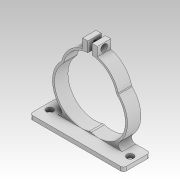
# Autodesk Inventor part: MotorTestBracket
Saved by Autodesk Inventor 2020 (Build 240168000, 168)
## iProperties
Created: 2022-01-15
Part Number: MotorTestBracket
Material: Generic
Document SubType Name: Modeling
Designer: DDeGo
Density: 1 g/cm^3
Appearance: Default
Author: DDeGo
Autodesk Inventor part; units mm, degrees
ref_plane "YZ Plane" through (0, 0, 0) normal (1, 0, 0) x (0, 1, 0)
ref_plane "XZ Plane" through (0, 0, 0) normal (0, 1, 0) x (-1, 0, 0)
ref_plane "XY Plane" through (0, 0, 0) normal (0, 0, 1) x (1, 0, 0)
sketch "Block1" plane through (0, 0, 0) normal (0, 0, 1) x (1, 0, 0)
  arc A0 (0.8192, -22.866) -> (-0.8192, -22.866) centre (0, -25.7519) ccw construction
  arc A1 (-20.2121, 10.7235) -> (-19.3929, 12.1424) centre (-22.3018, 12.876) ccw construction
  circle A2 centre (21.4359, -12.376) radius 1.25 construction
  circle A3 centre (22.4424, 3.0852) radius 1.25 construction
  arc A4 (0.8192, -22.866) -> (20.2121, 10.7235) centre (6.2805, -3.626) ccw construction
  circle A5 centre (-8.5493, -20.9783) radius 1.25 construction
  circle A6 centre (8.5493, -20.9783) radius 1.25 construction
  circle A7 centre (-22.4424, 3.0852) radius 1.25 construction
  arc A8 (-20.2121, 10.7235) -> (-0.8192, -22.866) centre (-6.2805, -3.626) ccw construction
  circle A9 centre (-21.4359, -12.376) radius 1.25 construction
  arc A10 (19.3929, 12.1424) -> (20.2121, 10.7235) centre (22.3018, 12.876) ccw construction
  arc A11 (19.3929, 12.1424) -> (-19.3929, 12.1424) centre (0, 7.2521) ccw construction
  circle A12 centre (-13.8931, 17.8931) radius 1.25 construction
  circle A13 centre (13.8931, 17.8931) radius 1.25 construction
  circle A14 centre (0, 24.7521) radius 1.25 construction
  arc A15 (19.5868, 12.1913) -> (-19.5868, 12.1913) centre (0, 7.2521) ccw
  arc A16 (19.5868, 12.1913) -> (20.3514, 10.867) centre (22.3018, 12.876) ccw
  arc A17 (0.7646, -23.0584) -> (20.3514, 10.867) centre (6.2805, -3.626) ccw
  arc A18 (0.7646, -23.0584) -> (-0.7646, -23.0584) centre (0, -25.7519) ccw
  arc A19 (-20.3514, 10.867) -> (-0.7646, -23.0584) centre (-6.2805, -3.626) ccw
  arc A20 (-20.3514, 10.867) -> (-19.5868, 12.1913) centre (-22.3018, 12.876) ccw
  arc A21 (0.355, -24.5013) -> (-0.355, -24.5013) centre (0, -25.7519) ccw
  arc A22 (0.355, -24.5013) -> (21.3963, 11.9432) centre (6.2805, -3.626) ccw
  arc A23 (21.0413, 12.5581) -> (21.3963, 11.9432) centre (22.3018, 12.876) ccw
  arc A24 (21.0413, 12.5581) -> (-21.0413, 12.5581) centre (0, 7.2521) ccw
  arc A25 (-21.3963, 11.9432) -> (-21.0413, 12.5581) centre (-22.3018, 12.876) ccw
  arc A26 (-21.3963, 11.9432) -> (-0.355, -24.5013) centre (-6.2805, -3.626) ccw
  line L0 (-5.5, 28.2435) -> (-5.5, 34.9521)
  line L1 (-5.5, 34.9521) -> (-1.5, 34.9521)
  line L2 (-1.5, 34.9521) -> (-1.5, 27.3963)
  line L3 (0, 24.7521) -> (0, 36.4403) construction
  line L4 (5.5, 28.2435) -> (5.5, 34.9521)
  line L5 (5.5, 34.9521) -> (1.5, 34.9521)
  line L6 (1.5, 34.9521) -> (1.5, 27.3963)
  point P0 (0, 0)
  dimension "d0" = 0.2
  dimension "d1" = 1.5
  dimension "d2" = 1.5
  dimension "d3" = 4
  dimension "d4" = 6
  measures "d0" radial gap between concentric circles of A11 A15
  measures "d1" radial gap between concentric circles of A19 A26
  measures "d2" distance between parallel lines of L2 L3
  measures "d3" distance of L0.end L1.end
  measures "d4" distance edge to line of A24 L1
sketch "Sketch2" plane through (0, 0, 0) normal (0, 0, 1) x (1, 0, 0)
  line L0 (-6.2805, -3.626) -> (0, 7.2521) construction
  line L1 (0, 7.2521) -> (6.2805, -3.626) construction
  line L2 (6.2805, -3.626) -> (-6.2805, -3.626) construction
  line L3 (-3.1402, 1.813) -> (0, 0) construction
  line L4 (0, 0) -> (3.1402, 1.813) construction
  line L5 (0, 0) -> (0, -3.626) construction
  arc A0 (0.8192, -22.866) -> (-0.8192, -22.866) centre (0, -25.7519) ccw construction
  arc A1 (-20.2121, 10.7235) -> (-19.3929, 12.1424) centre (-22.3018, 12.876) ccw construction
  circle A2 centre (21.4359, -12.376) radius 1.25 construction
  circle A3 centre (22.4424, 3.0852) radius 1.25 construction
  arc A4 (0.8192, -22.866) -> (20.2121, 10.7235) centre (6.2805, -3.626) ccw construction
  circle A5 centre (-8.5493, -20.9783) radius 1.25 construction
  circle A6 centre (8.5493, -20.9783) radius 1.25 construction
  circle A7 centre (-22.4424, 3.0852) radius 1.25 construction
  arc A8 (-20.2121, 10.7235) -> (-0.8192, -22.866) centre (-6.2805, -3.626) ccw construction
  circle A9 centre (-21.4359, -12.376) radius 1.25 construction
  arc A10 (19.3929, 12.1424) -> (20.2121, 10.7235) centre (22.3018, 12.876) ccw construction
  arc A11 (19.3929, 12.1424) -> (-19.3929, 12.1424) centre (0, 7.2521) ccw construction
  circle A12 centre (-13.8931, 17.8931) radius 1.25 construction
  circle A13 centre (13.8931, 17.8931) radius 1.25 construction
  circle A14 centre (0, 24.7521) radius 1.25 construction
  arc A15 (19.5868, 12.1913) -> (-19.5868, 12.1913) centre (0, 7.2521) ccw
  arc A16 (19.5868, 12.1913) -> (20.3514, 10.867) centre (22.3018, 12.876) ccw
  arc A17 (0.7646, -23.0584) -> (20.3514, 10.867) centre (6.2805, -3.626) ccw
  arc A18 (0.7646, -23.0584) -> (-0.7646, -23.0584) centre (0, -25.7519) ccw
  arc A19 (-20.3514, 10.867) -> (-0.7646, -23.0584) centre (-6.2805, -3.626) ccw
  arc A20 (-20.3514, 10.867) -> (-19.5868, 12.1913) centre (-22.3018, 12.876) ccw
  arc A21 (0.355, -24.5013) -> (-0.355, -24.5013) centre (0, -25.7519) ccw
  arc A22 (0.355, -24.5013) -> (21.3963, 11.9432) centre (6.2805, -3.626) ccw
  arc A23 (21.0413, 12.5581) -> (21.3963, 11.9432) centre (22.3018, 12.876) ccw
  arc A24 (21.0413, 12.5581) -> (-21.0413, 12.5581) centre (0, 7.2521) ccw
  arc A25 (-21.3963, 11.9432) -> (-21.0413, 12.5581) centre (-22.3018, 12.876) ccw
  arc A26 (-21.3963, 11.9432) -> (-0.355, -24.5013) centre (-6.2805, -3.626) ccw
  line L6 (-5.5, 28.2435) -> (-5.5, 34.9521)
  line L7 (-5.5, 34.9521) -> (-1.5, 34.9521)
  line L8 (-1.5, 34.9521) -> (-1.5, 27.3963)
  line L9 (0, 24.7521) -> (0, 36.4403) construction
  line L10 (5.5, 28.2435) -> (5.5, 34.9521)
  line L11 (5.5, 34.9521) -> (1.5, 34.9521)
  line L12 (1.5, 34.9521) -> (1.5, 27.3963)
  constraints: 12 end point, 3 coincident, 3 midpoint, 2 perpendicular, 1 horizontal, 3 other
extrude "Extrusion1" add sketch "Sketch2" along normal blind 10 contours A15 L12 A24 A23 A22 A21 A26 A25 L8 A20 A19 A18 A17 A16 | L12 L11 L10 A24 | A24 L6 L7 L8
sketch "Sketch3" plane through (5.5, 28.2435, 0) normal (1, 0, 0) x (0, 0, -1)
  line L0 (0, 6.7086) -> (-10, 6.7086) construction
  line L1 (-5, 6.7086) -> (-5, 0) construction
  line L2 (0, 0) -> (-10, 0) construction
  circle A0 centre (-5, 3.3543) radius 1.6
  point P0 (0, -28.2435)
  dimension "d7" = 3.2
  constraints: 3 midpoint, 2 end point, 1 centre point
  measures "d7" diameter of A0
extrude "Extrusion2" cut sketch "Sketch3" against normal through all
sketch "Sketch4" plane through (0, 0, 10) normal (0, 0, 1) x (1, 0, 0)
  line L0 (35, -26.826) -> (-35, -26.826)
  line L1 (-35, -26.826) -> (-35, -23.826)
  line L2 (-35, -23.826) -> (35, -23.826)
  line L3 (35, -23.826) -> (35, -26.826)
  arc A0 (-20.3514, 10.867) -> (-0.7646, -23.0584) centre (-6.2805, -3.626) ccw construction
  arc A1 (0.355, -24.5013) -> (-0.355, -24.5013) centre (0, -25.7519) ccw projected
  line L4 (0, -25.7519) -> (0, -23.826) construction
  point P0 (0, 0)
  dimension "d10" = 3
  dimension "d11" = 35
  dimension "d12" = 35
  constraints: 10 end point, 2 parallel, 2 perpendicular, 1 horizontal, 1 midpoint, 1 tangent
  measures "d10" distance between parallel lines of L0 L2
  measures "d11" distance between parallel lines of L4 L1
  measures "d12" distance between parallel lines of L3 L4
extrude "Extrusion3" add sketch "Sketch4" against normal up to surface (10 mm away)
fillet "Fillet1" radius 3 2 edges at (-14.2083, -23.826, 5) (14.2083, -23.826, 5)
sketch "Sketch6" plane through (0, 0, 10) normal (0, 0, 1) x (1, 0, 0)
  line L0 (-35, -26.826) -> (35, -26.826) projected
  line L1 (-35, -23.826) -> (-24.0076, -23.826) projected
  line L2 (35, -26.826) -> (-35, -26.826)
  line L3 (-35, -26.826) -> (-35, -23.826)
  line L4 (-35, -23.826) -> (35, -23.826)
  line L5 (35, -23.826) -> (35, -26.826)
  point P0 (0, 0)
  constraints: 8 end point, 2 parallel, 1 horizontal, 1 perpendicular
extrude "Extrusion5" add sketch "Sketch6" along normal blind 10
sketch "Sketch5" plane through (35, -23.826, 10) normal (0, 1, 0) x (1, 0, 0)
  line L0 (0, 0) -> (-5, 0) construction
  circle A0 centre (-5, 0) radius 2.6
  line L1 (-70, 0) -> (-65, 0) construction
  circle A1 centre (-65, 0) radius 2.6
  line L2 (0, 10) -> (0, -10) projected
  line L3 (-70, 10) -> (-70, -10) projected
  point P0 (-35, 10)
  dimension "d16" = 5
  dimension "d17" = 5.2
  constraints: 4 end point, 2 centre point, 2 coincident, 2 horizontal, 2 midpoint, 1 collinear, 1 equal radius
  measures "d16" distance of L0.start L0.end
  measures "d17" diameter of A0
extrude "Extrusion4" cut sketch "Sketch5" against normal blind 10
fillet "Fillet2" radius 2 4 edges at (35, -25.326, 0) (-35, -25.326, 0) (-35, -25.326, 20) (35, -25.326, 20)
sketch "Sketch7" plane through (5.5, 28.2435, 0) normal (1, 0, 0) x (0, 0, -1)
  circle A0 centre (-5, 3.3543) radius 1.6 projected
  circle A1 centre (-5, 3.3543) radius 2.54
  point P0 (0, -28.2435)
  dimension "d23" = 5.08
  constraints: 1 centre point, 1 coincident
  measures "d23" diameter of A1
extrude "Extrusion6" cut sketch "Sketch7" against normal up to surface (4 mm away) contours A0 | A1
equation "\"d12\" = d11"
body "Solid1"
